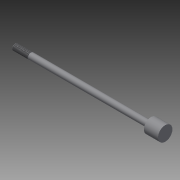
# Autodesk Inventor part: 012.5-DP0_rod
Saved by Autodesk Inventor 2015 (Build 190159000, 159)
## iProperties
Category: PARTsolutions
Company: BIMBA
Created: 2015-01-25
Part Number: 012.5-DP0_rod
Material: Generic
Catalog Web Link: www.cadenas.de
Description: Standard Air Cylinder_rod-Original Line - Standard Air Cylinders
Vendor: BIMBA
Document SubType Name: Standard Catalog Part
Designer: whitaus15
Manufacturer: BIMBA
Mass: 2.98336 g
Surface Area: 21.8044 cm^2
Volume: 2.98336 cm^3
Density: 1 g/cm^3
Appearance: PSOLRGB-181-181-181
PSOL_IDENT_0: {$CADENAS_DATA\23d-libs\bimba\bimba\bimba_imperial\bimba_full_line\original_line_cylinders\standard_
PSOL_IDENT_1: air_cylinders\rod.prj},280 {VTYP=3D},{NB=012.5-DP0_rod},{LINA=012.5-DP0_rod},{NN=Standard Air Cylind
PSOL_IDENT_2: er_rod},{DATE=08.09.2014 05:04:05},{GEOMDATE=08.09.2014 05:04:01},{VERSION=},{LINEID=30},{LINESUBID=
PSOL_IDENT_3: -1},{WBVAR=STROKE,ACTING,MNT,DER,NR,BM,CO,M,EE,EEL,K,Q,Y,F,G,T,B,H,SER,SR,NT,W,E,HL,ST,STP,PRC,PB,CO
PSOL_IDENT_4: LOR1}  {NB=012.5-DP0_rod},{LINA=012.5-DP0_rod},{KT=DUMMY},{PN=012.5-DP},{DASH=-},{BORE=0.43750000},{
PSOL_IDENT_5: BOREPN=01},{STROKE=2.500},{STROKEALG=[0.001:50/0.001]},{STROKE1=2.500},{ACTING=D},{ACTINGALG= '' , '
PSOL_IDENT_6: Single Acting' , 'R' , 'Reverse Single Acting' , 'D' , 'Double Acting' },{ACTINGPN=D},{MNT=P},{MNTAL
PSOL_IDENT_7: G= '' , 'Front Nose Mounting' , 'P' , 'Rear Pivot Mounting' , 'X' , 'Double End Mounting' , 'BF' , '
PSOL_IDENT_8: Front Block Mounting' , 'BR' , 'Rear Block Mounting for Vertical Positioning' , 'BFT' , 'Front Block
PSOL_IDENT_9: Trunnion Mounting' , 'BRT' , 'Rear Block Trunnion Mounting' },{TYPE=},{MNTPN=P},{DER=},{DERALG= ''
PSOL_IDENT_10: , 'N/A' },{NR=},{NRALG= '' , 'N/A' },{NRPN=},{BM=},{BMALG= '' , 'N/A' },{BMPN=},{CO=},{COALG= '' , '
PSOL_IDENT_11: N/A' },{M=},{MALG= '', 'Without Magnet', 'M', 'With Magnet' },{EE=},{EEL=0},{EEMAX=48},{EEALG= '', '
PSOL_IDENT_12: Without Extra Extension', 'EE', 'With Extra Extension' },{EELALG=0},{EEPN=},{EEPN1=0.000},{K=},{KALG=
PSOL_IDENT_13: '', 'Standard' , 'K' , 'Ports Rotated 90deg' },{KPN=},{Q=},{QALG= '' , 'Without Side Ported Rear He
PSOL_IDENT_14: ad' , 'Q' , 'With Side Ported Rear Head' },{QPN=},{Y=},{YALG= '' , 'Without Pivot Bushing' , 'Y' , '
PSOL_IDENT_15: With Pivot Bushing' },{YPN=},{F=},{FALG= '', 'Standard', 'F', 'Molycoated Body' },{FPN=},{G=},{GPN=}
PSOL_IDENT_16: ,{T=},{TALG= '' , 'Standard' , 'N' , 'Low Temperature' , 'V' , 'High Temperature' },{NPN=},{VPN=},{B=
PSOL_IDENT_17: },{BALG= '', 'Without Bumper' , 'B' , 'With Bumper' },{BPN=},{H=},{HALG= '', 'N/A' },{HPN=},{SER=},{
PSOL_IDENT_18: SERALG= '' , 'Without Spring Extend/Return' , 'JS' , 'With Spring Return' , 'JR' , 'With Spring Exte
PSOL_IDENT_19: nd' },{SR=},{SRALG= 'C' , 'Carbon Steel Rod' , 'SR' , '303 Stainless Steel Rod' , '' , '303 Stainles
PSOL_IDENT_20: s Steel Rod1' },{SRPN=},{SRCON=0},{NT=},{NTPN=},{W=},{WALG= '' , 'Without Wiper' , 'W' , 'With Wiper'
PSOL_IDENT_21: },{WPN=},{E=},{EALG= '' , 'Without Special Lube and Seals' , 'E' , 'With Special Lube and Seals' },
PSOL_IDENT_22: {EPN=},{HL=},{HLALG= '' , 'Wihout Low Pressure Hydraulic' , 'HL' , 'With Low Pressure Hydraulic' },{
PSOL_IDENT_23: ST=},{STALG= '' , 'Without Switch Track' , 'T' , 'With Switch Track' },{STP=},{STPALG= '' , 'N/A' },
PSOL_IDENT_24: {STPN=},{PRC=},{PRCALG= '' , 'Without Piston Rod Clevis' , 'D-166-1' , 'With Piston Rod Clevis' },{P
PSOL_IDENT_25: RCPN=},{PB=},{PBALG= '' , 'Without Pivot Bracket' , 'D-167' , 'With Pivot Bracket' },{PBPN=},{TLEN=3
PSOL_IDENT_26: .2700},{TEXT=0.266667},{SPACE=0.152381},{FRAC=15.0600},{RGCON=},{RGDACCON=R},{RHCON=P},{RHCONON=1},{
PSOL_IDENT_27: RHACCON=R},{FNUTCON=0},{RNUTCON=0},{FNUTPN=},{RNUTPN=},{FNUTTRANS=0.0000},{RNUTTRANS=0.0000},{VHOLEC
PSOL_IDENT_28: ON=0},{A1=1.1880},{A1N=0.6880},{A1P=1.1880},{A1B=1.1880},{A4=0.1880},{A4N=0.2500},{A4P=0.1880},{A5=0
PSOL_IDENT_29: .0200},{A1H=1.188},{A1NH=0.5000},{A1PH=1.1880},{A1BH=0.8120},{A1SH=0.0000},{A2H=0.1880},{A2NH=0.1880
PSOL_IDENT_30: },{LENGTH=2.5600},{LENGTH1=2.5600},{LENGTH2=2.6100},{MUL=2.5000},{MUL11=2.5000},{MUL22=7.2000},{MUL3
PSOL_IDENT_31: 3=4.7000},{MUL2=2.5000},{MUL211=2.5000},{MUL222=1.4400},{MUL233=0.9400},{SSS=5.0000},{RGLEN=1.0200},
PSOL_IDENT_32: {RHLEN=0.7700},{SSS1=5.0000},{A13=0.9380},{THDLEN1=0.5000},{THD1=0.1900},{TAB=UNF},{THDLEN=0.5000},{
PSOL_IDENT_33: THD=0.1900},{OD=0.4465},{RODL=4.6220},{PL=0.4340},{RODDIA=0.1870},{HEX=0.1870},{RODTRANS=0.0000},{G1=
PSOL_IDENT_34: 0.0000},{ON=0},{G5=0.0000},{DERLEN=4.1880},{THOLE=0.0000},{WF=0.0000},{BADD=0.0000},{MADD=0.0000},{N
PSOL_IDENT_35: VADD=0.000},{JRADD=0.00000},{COLOR=0.71,0.71,0.71,0.00},{GROOVE=1},{HOL=0},{D7=0.1590},{H1=0.0000},{
PSOL_IDENT_36: D1=0.7380},{D1RH=0.7380},{D1P=0.0000},{D1B=0.7380},{D1N=0.4840},{D1NRH=0.4855},{D1BRH=0.4855},{D1PRH=
PSOL_IDENT_37: 0.7380},{BOZO=0},{HADD=0.000},{COLOR1=0},{DEFL=0.0000},{HEXL=0.0000},{SSADD=0.0000},{WFL=0.0000},{MO
PSOL_IDENT_38: VE=0.0000},{PRCL2=0.37500},{PRCB=0.12000},{PRCTRANS=0.00000}
NN: Standard Air Cylinder_rod
NT: Standard
NB: 012.5-DP0_rod
NBSYN: $PN.$COLOR1._rod
LINA: 012.5-DP0_rod
PN: 012.5-DP
BORE: 0.43750000
BOREPN: 01
STROKE: 2.500
ACTING: Double Acting
MNT: Rear Pivot Mounting
DER: N/A
NR: N/A
BM: N/A
CO: N/A
M: Without Magnet
EE: Without Extra Extension
EEL: 0
K: Standard
Q: Without Side Ported Rear Head
Y: Without Pivot Bushing
F: Standard
G: Without Magnalube Lubrication
T: Standard
B: Without Bumper
H: N/A
SER: Without Spring Extend/Return
SR: 303 Stainless Steel Rod1
W: Without Wiper
E: Without Special Lube and Seals
HL: Wihout Low Pressure Hydraulic
ST: Without Switch Track
STP: N/A
PRC: Without Piston Rod Clevis
PB: Without Pivot Bracket
A1N: 0.6880
A1P: 1.1880
A1B: 1.1880
A4N: 0.2500
A4P: 0.1880
A5: 0.0200
A1NH: 0.5000
A1PH: 1.1880
A1BH: 0.8120
A1SH: 0.0000
A2NH: 0.1880
A13: 0.9380
THDLEN1: 0.5000
THD1: 0.1900
TAB: UNF
OD: 0.4465
RODDIA: 0.1870
HEX: 0.1870
G1: 0.0000
G5: 0.0000
THOLE: 0.0000
WF: 0.0000
GROOVE: 1
D7: 0.1590
D1P: 0.0000
D1B: 0.7380
D1N: 0.4840
D1NRH: 0.4855
D1BRH: 0.4855
D1PRH: 0.7380
COLOR1: 0
SUPPLIER: BIMBA
ARTICLENO: 012.5-DP0_rod
BOMINFO: 012.5-DP0_rod
CREATOR: CADENAS GmbH
Title: 012.5-DP0_rod
Author: Cadenas PARTsolutions
Comments: Original Line - Standard Air Cylinders
Autodesk Inventor part; units mm, degrees
sketch "Sketch_1" plane through (0, 0, 0) normal (0, 0, 1) x (1, 0, 0)
  line L0 (104.6988, 0) -> (0, 0)
  line L1 (0, 0) -> (0, 2.3749)
  line L2 (0, 2.3749) -> (93.6752, 2.3749)
  line L3 (93.6752, 2.3749) -> (93.6752, 5.6197)
  line L4 (93.6752, 5.6197) -> (104.6988, 5.6197)
  line L5 (104.6988, 5.6197) -> (104.6988, 0)
  line L6 (104.6988, 0) -> (0, 0)
  constraints: 14 end point
revolve "Revolution1" add sketch "Sketch_1" angle 360 about axis through (104.6988, 0, 0) along (1, 0, 0)
sketch "Sketch_3" plane through (0, 0, 0) normal (0, 0, 1) x (1, 0, 0)
  line L0 (0, 0) -> (-12.7, 0)
  line L1 (-12.7, 0) -> (-12.7, 1.9406)
  line L2 (-12.7, 1.9406) -> (-12.2276, 2.413)
  line L3 (-12.2276, 2.413) -> (0, 2.413)
  line L4 (0, 2.413) -> (0, 0)
  line L5 (0, 0) -> (-12.7, 0)
  constraints: 12 end point
revolve "Revolution2" add sketch "Sketch_3" angle 360 about axis through (0, 0, 0) along (1, 0, 0)
thread "Thread1" size "10-32 UNF" class "2A" standard "ANSI Unified Screw Threads" full length
sketch "Sketch_30" plane through (0, 0, 0) normal (0, 0, 1) x (1, 0, 0)
  line L0 (0, 0) -> (-0.254, 0)
  line L1 (-0.254, 2.667) -> (-0.254, 2.159)
  line L2 (-0.254, 2.159) -> (0, 2.159)
  line L3 (0, 2.159) -> (0, 2.667)
  line L4 (0, 2.667) -> (-0.254, 2.667)
  constraints: 10 end point
revolve "Revolution3" cut sketch "Sketch_30" angle 360 about axis through (0, 0, 0) along (1, 0, 0)
ref_plane "dia1_XY" through (0, 2.3749, 0) normal (1, 0, 0) x (0, 0, -1)
ref_plane "dia1_YZ" through (0, 2.3749, 0) normal (0, 0, -1) x (0, 1, 0)
ref_plane "dia1_ZX" through (0, 2.3749, 0) normal (0, 1, 0) x (1, 0, 0)
ref_plane "dia12_XY" through (0, 0, 9.3726) normal (1, 0, 0) x (0, 0, -1)
ref_plane "dia12_YZ" through (0, 0, 9.3726) normal (0, 0, -1) x (0, 1, 0)
ref_plane "dia12_ZX" through (0, 0, 9.3726) normal (0, 1, 0) x (1, 0, 0)
ref_plane "dia2_XY" through (0, -2.3749, 0) normal (1, 0, 0) x (0, 0, -1)
ref_plane "dia2_YZ" through (0, -2.3749, 0) normal (0, 0, -1) x (0, 1, 0)
ref_plane "dia2_ZX" through (0, -2.3749, 0) normal (0, 1, 0) x (1, 0, 0)
ref_plane "dia22_XY" through (0, 0, -9.3726) normal (1, 0, 0) x (0, 0, -1)
ref_plane "dia22_YZ" through (0, 0, -9.3726) normal (0, 0, -1) x (0, 1, 0)
ref_plane "dia22_ZX" through (0, 0, -9.3726) normal (0, 1, 0) x (1, 0, 0)
ref_plane "rl1_XY" through (-12.7, 0, 0) normal (1, 0, 0) x (0, 0, -1)
ref_plane "rl1_YZ" through (-12.7, 0, 0) normal (0, 0, -1) x (0, 1, 0)
ref_plane "rl1_ZX" through (-12.7, 0, 0) normal (0, 1, 0) x (1, 0, 0)
ref_plane "rl2_XY" through (0, 0, 0) normal (1, 0, 0) x (0, 0, -1)
ref_plane "rl2_YZ" through (0, 0, 0) normal (0, 0, -1) x (0, 1, 0)
ref_plane "rl2_ZX" through (0, 0, 0) normal (0, 1, 0) x (1, 0, 0)
ref_plane "rod_cp_XY" through (0, 0, 0) normal (1, 0, 0) x (0, 0, -1)
ref_plane "rod_cp_YZ" through (0, 0, 0) normal (0, 0, -1) x (0, 1, 0)
ref_plane "rod_cp_ZX" through (0, 0, 0) normal (0, 1, 0) x (1, 0, 0)
ref_plane "thd1_XY" through (-12.7, 2.413, 0) normal (1, 0, 0) x (0, 0, -1)
ref_plane "thd1_YZ" through (-12.7, 2.413, 0) normal (0, 0, -1) x (0, 1, 0)
ref_plane "thd1_ZX" through (-12.7, 2.413, 0) normal (0, 1, 0) x (1, 0, 0)
ref_plane "thd2_XY" through (-12.7, -2.413, 0) normal (1, 0, 0) x (0, 0, -1)
ref_plane "thd2_YZ" through (-12.7, -2.413, 0) normal (0, 0, -1) x (0, 1, 0)
ref_plane "thd2_ZX" through (-12.7, -2.413, 0) normal (0, 1, 0) x (1, 0, 0)
ref_plane "to_rod_clevis_XY" through (-12.7, 0, 0) normal (1, 0, 0) x (0, 0, -1)
ref_plane "to_rod_clevis_YZ" through (-12.7, 0, 0) normal (0, 0, -1) x (0, 1, 0)
ref_plane "to_rod_clevis_ZX" through (-12.7, 0, 0) normal (0, 1, 0) x (1, 0, 0)
body "Solid1"
